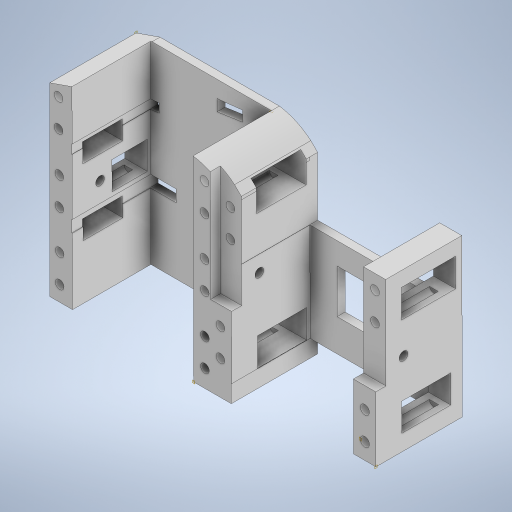
# Autodesk Inventor part: plaque motor
Saved by Autodesk Inventor 2024 (Build 280153000, 153)
## iProperties
Created: 2025-06-26
Part Number: plaque motor
Material: Generic
Document SubType Name: Modeling
Designer: Mehdi Charfeddine
Density: 1 g/cm^3
Appearance: Default
Author: Mehdi Charfeddine
Autodesk Inventor part; units mm, degrees
ref_plane "YZ Plane" through (0, 0, 0) normal (1, 0, 0) x (0, 1, 0)
ref_plane "XZ Plane" through (0, 0, 0) normal (0, 1, 0) x (-1, 0, 0)
ref_plane "XY Plane" through (0, 0, 0) normal (0, 0, 1) x (1, 0, 0)
ref_plane "Work Plane1" through (-1254.3029, 331.2668, 0) normal (0, 0, -1) x (-1, 0, 0)
sketch "Sketch1" plane through (-1254.3029, 331.2668, 0) normal (0, 0, -1) x (-1, 0, 0)
  line L0 (143.493, -1179.4126) -> (-2698.903, -1179.4126)
  line L1 (-2698.903, -1179.4126) -> (-2698.903, 519.8008)
  line L2 (-2698.903, 519.8008) -> (143.493, 519.8008)
  line L3 (143.493, 519.8008) -> (143.493, -1179.4126)
  line L4 (143.493, -1161.471) -> (-468.5573, -1161.471)
  line L5 (-468.5573, -1161.471) -> (-468.5573, -1017.271)
  line L6 (-468.5573, -1017.271) -> (-637.164, -1026.0298)
  line L7 (-637.164, -1026.0298) -> (-1102.7998, -1026.0298)
  line L8 (-1102.7998, -1026.0298) -> (-1102.7998, -1179.4126)
  line L9 (-1434.9695, -1179.4126) -> (-1434.9695, -1026.0298)
  line L10 (-1434.9695, -1026.0298) -> (-2698.903, -1026.0298)
  line L11 (-2496.2093, 337.6122) -> (-2698.903, 337.6122)
  line L12 (-2496.2093, 337.6122) -> (-2496.2093, -173.286)
  line L13 (-2496.2093, -173.286) -> (-1434.9695, -173.286)
  line L14 (-1434.9695, -173.286) -> (-1434.9695, 337.6122)
  line L15 (-1434.9695, 337.6122) -> (-1234.6616, 535.9778)
  line L16 (173.3581, 436.795) -> (-144.8352, 547.7469)
  line L17 (-1673.6533, -745.0956) -> (-1673.6533, -364.1105)
  line L18 (-1673.6533, -364.1105) -> (-2283.8134, -364.1105)
  line L19 (-2283.8134, -364.1105) -> (-2283.8134, -745.0956)
  line L20 (-2283.8134, -745.0956) -> (-1673.6533, -745.0956)
  line L21 (-685.7764, -398.0133) -> (-685.7764, -278.9407)
  line L22 (-685.7764, -278.9407) -> (-851.0206, -278.9407)
  line L23 (-851.0206, -278.9407) -> (-851.0206, -398.0133)
  line L24 (-851.0206, -398.0133) -> (-685.7764, -398.0133)
  line L25 (-47.919, -587.3066) -> (-47.6877, -587.3066)
  line L26 (-47.6877, -587.3066) -> (-47.6877, -483.7142)
  line L27 (-47.6877, -483.7142) -> (-47.919, -483.7142)
  line L28 (-47.919, -483.7142) -> (-47.919, -587.3066)
  line L29 (-274.0649, -587.3066) -> (-47.6877, -587.3066)
  line L30 (-47.6877, -587.3066) -> (-47.6877, -483.7142)
  line L31 (-47.6877, -483.7142) -> (-274.0649, -483.7142)
  line L32 (-274.0649, -483.7142) -> (-274.0649, -587.3066)
  line L33 (-47.6806, 4.4603) -> (-47.6806, 82.2285)
  line L34 (-47.6806, 82.2285) -> (-125.767, 90.6905)
  line L35 (-125.767, 90.6905) -> (-125.767, 12.9223)
  line L36 (-125.767, 12.9223) -> (-47.6806, 4.4603)
  line L37 (-630.1703, 275.0879) -> (-630.1703, 374.6704)
  line L38 (-630.1703, 374.6704) -> (-851.0206, 398.6035)
  line L39 (-851.0206, 398.6035) -> (-851.0206, 307.8079)
  line L40 (-851.0206, 307.8079) -> (-630.1703, 275.0879)
  point P0 (-1254.3029, -331.2668)
  point P1 (143.493, 447.2087)
  point P2 (-64.69, 519.8008)
  point P3 (-1250.997, 519.8008)
  constraints: 82 end point, 15 perpendicular, 12 parallel, 9 point on line, 5 vertical, 3 horizontal
extrude "Extrusion1" add sketch "Sketch1" against normal blind 1100 contours L0 L9 L10 L1 L11 L12 L13 L14 L15 L2 L16 L3 L4 L5 L6 L7 L8
ref_plane "Work Plane2" through (-149.2504, 846.8869, 69.2404) normal (-0.0030203, 0.9999954, 0) x (-0.9999954, -0.0030203, 0)
sketch "Sketch3" plane through (-149.2504, 846.8869, 69.2404) normal (-0.0030203, 0.9999954, 0) x (-0.9999954, -0.0030203, 0)
  line L0 (-1582.4068, 681.0018) -> (-1388.0405, 681.0018)
  line L1 (-1388.0405, 681.0018) -> (-1388.0405, -0.3135)
  line L2 (-1388.0405, -0.3135) -> (-329.2978, -0.3135)
  line L3 (-329.2978, -0.3135) -> (-329.2978, 936.8883)
  line L4 (-329.2978, 936.8883) -> (-146.6919, 936.8883)
  line L5 (-146.6919, 936.8883) -> (-146.6919, 681.0018)
  line L6 (-146.6919, 681.0018) -> (2.4104, 681.0018)
  line L7 (2.4104, 681.0018) -> (2.4104, -0.3135)
  line L8 (2.4104, -0.3135) -> (1055.5167, -0.3135)
  line L9 (1055.5167, -0.3135) -> (1055.5167, 681.0018)
  line L10 (1055.5167, 681.0018) -> (1255.081, 681.0018)
  line L11 (1255.081, 681.0018) -> (1255.081, -69.2404)
  line L12 (1255.081, -69.2404) -> (-1582.4068, -69.2404)
  line L13 (-1582.4068, -69.2404) -> (-1582.4068, 681.0018)
  line L14 (-1708.3314, 1095.6813) -> (1374.7407, 1095.6813)
  line L15 (1374.7407, 1095.6813) -> (1374.7407, -238.0329)
  line L16 (1374.7407, -238.0329) -> (-1708.3314, -238.0329)
  line L17 (-1708.3314, -238.0329) -> (-1708.3314, 1095.6813)
  point P0 (-146.6919, -69.2404)
  constraints: 36 end point, 11 perpendicular, 6 point on line, 2 horizontal, 2 parallel
extrude "Extrusion2" cut sketch "Sketch3" along normal through all both and the other way through all
ref_plane "Work Plane3" through (1301.039, -554.482, 749.7064) normal (0, 0, 1) x (1, 0, 0)
sketch "Sketch5" plane through (1301.039, -554.482, 749.7064) normal (0, 0, 1) x (1, 0, 0)
  circle A0 centre (40.4282, 0.3017) radius 39.6541
  circle A1 centre (40.4282, 242.0442) radius 39.2588
  circle A2 centre (40.4282, 855.1691) radius 38.244
  circle A3 centre (40.4282, 1097.0764) radius 37.9245
  circle A4 centre (-1215.2062, 242.0442) radius 37.5
  circle A5 centre (-1351.3818, 438.4816) radius 37.5
  circle A6 centre (-1349.8368, -141.9533) radius 37.5
  circle A7 centre (-1215.2062, 0.3017) radius 37.5
  circle A8 centre (-1349.8368, 97.9228) radius 37.5
  circle A9 centre (-1352.711, 680.6295) radius 37.5
  circle A10 centre (-1215.2062, 855.1691) radius 37.5
  circle A11 centre (-1215.2062, 1097.0764) radius 37.5
  circle A12 centre (-1352.711, 1024.6066) radius 37.5
  circle A13 centre (-1352.711, 1266.5769) radius 37.5
  circle A14 centre (-2612.1591, -141.9533) radius 37.5
  circle A15 centre (-2612.1591, 100.2141) radius 37.5
  circle A16 centre (-2615.3984, 438.4816) radius 37.5
  circle A17 centre (-2615.3984, 680.6295) radius 37.5
  circle A18 centre (-2621.8923, 1024.6066) radius 37.5
  circle A19 centre (-2621.8923, 1266.5769) radius 37.5
  point P0 (-1301.039, 554.482)
  dimension "d5" = 75
  dimension "d6" = 75
  dimension "d7" = 75
  dimension "d8" = 75
  dimension "d9" = 75
  dimension "d10" = 75
  dimension "d11" = 75
  dimension "d12" = 75
  dimension "d13" = 75
  dimension "d14" = 75
  dimension "d15" = 75
  dimension "d16" = 75
  dimension "d17" = 75
  dimension "d18" = 75
  dimension "d19" = 75
  dimension "d20" = 75
  constraints: 20 centre point
  measures "d5" diameter of A4
  measures "d6" diameter of A5
  measures "d7" diameter of A6
  measures "d8" diameter of A7
  measures "d9" diameter of A8
  measures "d10" diameter of A9
  measures "d11" diameter of A10
  measures "d12" diameter of A11
  measures "d13" diameter of A12
  measures "d14" diameter of A13
  measures "d15" diameter of A14
  measures "d16" diameter of A15
  measures "d17" diameter of A16
  measures "d18" diameter of A17
  measures "d19" diameter of A18
  measures "d20" diameter of A19
ref_plane "Work Plane4" through (-149.2504, 846.8869, 69.2404) normal (-0.0030203, 0.9999954, 0) x (-0.9999954, -0.0030203, 0)
sketch "Sketch6" plane through (-149.2504, 846.8869, 69.2404) normal (-0.0030203, 0.9999954, 0) x (-0.9999954, -0.0030203, 0)
  line L0 (-327.1377, 938.1935) -> (-146.6919, 938.1935)
  line L1 (-146.6919, 938.1935) -> (-146.6919, 593.8653)
  line L2 (-146.6919, 593.8653) -> (-327.1377, 593.8653)
  line L3 (-327.1377, 593.8653) -> (-327.1377, 938.1935)
  line L4 (-146.6919, 593.8653) -> (-382.456, 593.8653)
  line L5 (-382.456, 593.8653) -> (-382.456, 1000.2855)
  line L6 (-382.456, 1000.2855) -> (-146.6919, 1000.2855)
  line L7 (-146.6919, 1000.2855) -> (-146.6919, 593.8653)
  point P0 (-146.6919, -69.2404)
  point P1 (-146.6919, 938.1935)
  constraints: 16 end point, 4 parallel, 2 horizontal, 2 perpendicular
extrude "Extrusion3" cut sketch "Sketch6" against normal blind 1000
sketch "Sketch7" plane through (1241.9064, 668.879, 0) normal (0, 1, 0) x (1, 0, 0)
  line L0 (-20.5264, -772.7264) -> (215.0683, -772.7264)
  line L1 (215.0683, -772.7264) -> (215.0683, -661.6695)
  line L2 (215.0683, -661.6695) -> (-20.5264, -661.6695)
  line L3 (-20.5264, -661.6695) -> (-20.5264, -772.7264)
  point P0 (-1241.9064, 0)
  constraints: 8 end point, 2 parallel, 1 horizontal, 1 perpendicular
extrude "Extrusion4" cut sketch "Sketch7" against normal blind 800
sketch "Sketch8" plane through (180.6666, -694.763, 0) normal (0, -1, 0) x (1, 0, 0)
  line L0 (1279.9894, 750.2422) -> (-280.5471, 750.2422)
  line L1 (-280.5471, 750.2422) -> (-280.5471, 1145.0076)
  line L2 (-280.5471, 1145.0076) -> (1279.9894, 1145.0076)
  line L3 (1279.9894, 1145.0076) -> (1279.9894, 750.2422)
  point P0 (-180.6666, 0)
  constraints: 8 end point, 2 parallel, 1 horizontal, 1 perpendicular
extrude "Extrusion5" cut sketch "Sketch8" along normal mid plane 1200
ref_plane "Work Plane5" through (-1397.762, 778.8657, 0) normal (-1, 0, 0) x (0, -1, 0)
sketch "Sketch9" plane through (-1397.762, 778.8657, 0) normal (-1, 0, 0) x (0, -1, 0)
  line L0 (395.7069, 657.3349) -> (559.2274, 657.3349)
  line L1 (559.2274, 657.3349) -> (559.2274, 311.254)
  line L2 (559.2274, 311.254) -> (395.7069, 311.254)
  line L3 (395.7069, 311.254) -> (395.7069, 657.3349)
  line L4 (975.9507, 657.3349) -> (1137.4736, 657.3349)
  line L5 (1137.4736, 657.3349) -> (1137.4736, 311.254)
  line L6 (1137.4736, 311.254) -> (975.9507, 311.254)
  line L7 (975.9507, 311.254) -> (975.9507, 657.3349)
  line L8 (653.2284, 98.0679) -> (895.5408, 98.0679)
  line L9 (895.5408, 98.0679) -> (895.5408, 404.469)
  line L10 (895.5408, 404.469) -> (653.2284, 404.469)
  line L11 (653.2284, 404.469) -> (653.2284, 98.0679)
  circle A0 centre (760.9225, 508.8229) radius 37.5
  point P0 (778.8657, 0)
  dimension "d27" = 75
  constraints: 24 end point, 6 parallel, 3 horizontal, 3 perpendicular, 2 point on line, 1 centre point
  measures "d27" diameter of A0
extrude "Extrusion6" cut sketch "Sketch9" along normal mid plane 1200
sketch "Sketch10" plane through (-151.6735, 851.0676, 68.9269) normal (-0.9999954, -0.0030203, 0) x (0, 0, 1)
  line L0 (456.3862, -1545.8838) -> (30.344, -1545.8838)
  line L1 (30.344, -1545.8838) -> (30.344, -1299.136)
  line L2 (30.344, -1299.136) -> (456.3862, -1299.136)
  line L3 (456.3862, -1299.136) -> (456.3862, -1545.8838)
  line L4 (463.9231, -135.8433) -> (30.344, -135.8433)
  line L5 (30.344, -135.8433) -> (30.344, -378.6799)
  line L6 (30.344, -378.6799) -> (463.9231, -378.6799)
  line L7 (463.9231, -378.6799) -> (463.9231, -135.8433)
  point P0 (-68.9269, -851.5219)
  constraints: 16 end point, 4 parallel, 2 horizontal, 2 perpendicular
extrude "Extrusion7" cut sketch "Sketch10" along normal mid plane 1200
ref_plane "Work Plane7" through (1437.8199, -694.763, 750.2422) normal (0.9999954, 0.0030203, 0) x (0, 0, -1)
sketch "Sketch11" plane through (1437.8199, -694.763, 750.2422) normal (0.9999954, 0.0030203, 0) x (0, 0, -1)
  line L0 (650.9713, 4.7405) -> (650.9713, 251.4883) projected
  line L1 (650.9713, 139.8075) -> (224.3628, 139.8075)
  line L2 (224.3628, 139.8075) -> (224.3628, 381.3673)
  line L3 (224.3628, 381.3673) -> (650.9713, 381.3673)
  line L4 (650.9713, 381.3673) -> (650.9713, 139.8075)
  line L5 (695.9796, 991.0182) -> (224.3628, 991.0182)
  line L6 (224.3628, 991.0182) -> (224.3628, 1236.4123)
  line L7 (224.3628, 1236.4123) -> (695.9796, 1236.4123)
  line L8 (695.9796, 1236.4123) -> (695.9796, 991.0182)
  point P0 (750.2422, 699.1025)
  constraints: 16 end point, 4 parallel, 2 horizontal, 2 perpendicular, 2 point on line
extrude "Extrusion8" cut sketch "Sketch11" along normal mid plane 1200
extrude "Extrusion9" cut sketch "Sketch5" along normal mid plane 1200
ref_plane "Work Plane6" through (-146.5413, -848.1458, 750.2422) normal (0, 0, 1) x (1, 0, 0)
sketch "Sketch12" plane through (-146.5413, -848.1458, 750.2422) normal (0, 0, 1) x (1, 0, 0)
  line L0 (327.1276, 1517.1043) -> (327.2078, 1490.531) projected
  line L1 (0, 0) -> (-5.1322, 1699.2134) projected
  arc A0 (327.1276, 1517.1043) -> (-5.1322, 1699.2134) centre (-83.8907, 1161.3577) ccw
  arc A1 (327.1276, 1517.1043) -> (-5.1322, 1699.2134) centre (180.0421, 1642.9056) ccw
  point P0 (146.5413, 848.1458)
  constraints: 4 point on circle, 2 centre point
extrude "Extrusion10" cut sketch "Sketch12" along normal through all both and the other way through all
sketch "Sketch13" plane through (-1397.7959, -830.2042, 0) normal (-1, 0, 0) x (0, 0, 1)
  circle A0 centre (508.8229, 848.1474) radius 37.5 projected
  circle A1 centre (508.8229, 848.1474) radius 37.5
  point P0 (0, 830.2042)
  constraints: 1 centre point, 1 coincident
extrude "Extrusion11" cut sketch "Sketch13" along normal through all both and the other way through all
sketch "Sketch14" plane through (-1397.7959, -830.2042, 0) normal (-1, 0, 0) x (0, 0, 1)
  point P0 (0, 830.2042)
body "Solid1"
